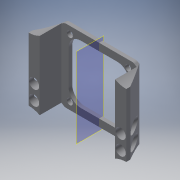
# Autodesk Inventor part: 30mm_fan_plus_radial
Saved by Autodesk Inventor 2019 (Build 230136000, 136)
## iProperties
Created: 2020-05-27
Part Number: 30mm_fan_plus_radial
Material: Generisch
Document SubType Name: Modeling
Designer: marc
Density: 1 g/cm^3
Appearance: Vorgabe
Author: marc
Autodesk Inventor part; units mm, degrees
ref_plane "YZ Plane" through (0, 0, 0) normal (1, 0, 0) x (0, 1, 0)
ref_plane "XZ Plane" through (0, 0, 0) normal (0, 1, 0) x (-1, 0, 0)
ref_plane "XY Plane" through (0, 0, 0) normal (0, 0, 1) x (1, 0, 0)
sketch "Skizze1" plane through (0, 0, 0) normal (0, 0, 1) x (1, 0, 0)
  arc A0 (-11.0395, 12.8) -> (-12.9605, 12.8) centre (-12, 12) ccw projected
  arc A1 (-12.9605, 11.2) -> (-11.0395, 11.2) centre (-12, 12) ccw projected
  arc A2 (-11.0395, -11.2) -> (-12.9605, -11.2) centre (-12, -12) ccw projected
  arc A3 (-12.9605, -12.8) -> (-11.0395, -12.8) centre (-12, -12) ccw projected
  arc A4 (12.9605, 12.8) -> (11.0395, 12.8) centre (12, 12) ccw projected
  arc A5 (11.0395, 11.2) -> (12.9605, 11.2) centre (12, 12) ccw projected
  arc A6 (11.0395, -12.8) -> (12.9605, -12.8) centre (12, -12) ccw projected
  arc A7 (12.9605, -11.2) -> (11.0395, -11.2) centre (12, -12) ccw projected
  line L0 (-13.5, 15) -> (13.5, 15)
  line L1 (15.5, 13) -> (15.5, -13)
  line L2 (13.5, -15) -> (-13.5, -15)
  line L3 (-15.5, -13) -> (-15.5, 13)
  arc A8 (-15.5, -13) -> (-13.5, -15) centre (-13.5, -13) ccw
  arc A9 (-13.5, 15) -> (-15.5, 13) centre (-13.5, 13) ccw
  arc A10 (15.5, 13) -> (13.5, 15) centre (13.5, 13) ccw
  arc A11 (13.5, -15) -> (15.5, -13) centre (13.5, -13) ccw
  line L4 (-7.5, -12) -> (7.5, -12)
  line L5 (12.5, -7) -> (12.5, 7)
  line L6 (7.5, 12) -> (-7.5, 12)
  line L7 (-12.5, 7) -> (-12.5, -7)
  arc A12 (-7.5, 12) -> (-12.5, 7) centre (-7.5, 7) ccw
  arc A13 (12.5, 7) -> (7.5, 12) centre (7.5, 7) ccw
  arc A14 (7.5, -12) -> (12.5, -7) centre (7.5, -7) ccw
  arc A15 (-12.5, -7) -> (-7.5, -12) centre (-7.5, -7) ccw
  circle A16 centre (-12, -12) radius 1.25
  circle A17 centre (12, 12) radius 1.25
  circle A18 centre (12, -12) radius 1.25
  circle A19 centre (-12, 12) radius 1.25
  point P0 (0, 0)
  point P1 (15.5, -15)
  point P2 (15.5, 15)
  point P3 (-15.5, -15)
  dimension "d0" = 31
  dimension "d1" = 30
  dimension "d2" = 3.5
  dimension "d3" = 3
  dimension "d4" = 2
  dimension "d5" = 5
  dimension "d6" = 5
  dimension "d7" = 3
  dimension "d8" = 3
  dimension "d9" = 3
  dimension "d10" = 3
  constraints: 16 end point, 16 point on circle, 16 tangent, 10 centre point, 7 equal radius, 6 point on line, 4 coincident, 4 parallel, 2 horizontal, 2 perpendicular, 6 other
  measures "d0" distance of point (15.5, -15) point (-15.5, -15)
  measures "d1" distance of point (15.5, 15) point (15.5, -15)
  measures "d2" distance from line of L3 A3.centre
  measures "d3" distance from line of L2 A2.centre
  measures "d4" radius of A8
  measures "d5" radius of A12
  measures "d6" radius of A13
  measures "d7" distance between parallel lines of L0 L6
  measures "d8" distance between parallel lines of L3 L7
  measures "d9" distance between parallel lines of L1 L5
  measures "d10" distance between parallel lines of L2 L4
extrude "Extrusion1" add sketch "Skizze1" along normal blind 1.5
sketch "Skizze2" plane through (15.5, -13, 0) normal (1, 0, 0) x (0, 0, -1)
  line L0 (0, 26) -> (-10.4, 26)
  line L1 (-10.4, 26) -> (-10.4, 0)
  line L2 (-10.4, 0) -> (0, 0)
  line L3 (0, 0) -> (0, 26)
  line L4 (0, 26) -> (-1.5, 26) projected
  point P0 (0, 13)
  dimension "d13" = 10.4
  constraints: 8 end point, 2 parallel, 1 coincident, 1 horizontal, 1 perpendicular
  measures "d13" distance of L1.end L2.end
extrude "Extrusion2" add sketch "Skizze2" along normal blind 4.6
chamfer "Fase1" distance 8.75 angle 25 1 edges at (20.1, 0, 0) measured on face at (20.1, 4.3333, 6.9333)
fillet "Rundung1" radius 9.75 1 edges at (15.5, -13, 0.75)
fillet "Rundung2" radius 9.75 1 edges at (15.5, 13, 0.75)
sketch "Skizze3" plane through (20.1, -13, 10.4) normal (0, 0, 1) x (1, 0, 0)
  line L0 (0, 26) -> (0, 0) projected
  line L1 (-4.6, -1.1307) -> (-4.6, 27.1307) projected
  point P0 (-20.1, 13)
  point P1 (-2.3, 9)
  point P2 (-2.3, 3)
  dimension "d21" = 2.3
  dimension "d22" = 4.6
  dimension "d23" = 3
  dimension "d24" = 6
  constraints: 1 vertical alignment
  measures "d21" distance from line of L0 point (-2.3, 3)
  measures "d22" distance between parallel lines of L0 L1
  measures "d23" vertical distance of L0.end point (-2.3, 3)
  measures "d24" distance of point (-2.3, 9) point (-2.3, 3)
hole "Bohrung1" at (17.8, -4, 10.4) at (17.8, -10, 10.4) direction (0, 0, -1) diameter 4.2 end through all
ref_plane "Arbeitsebene1" through (0, -13, 0) normal (-1, 0, 0) x (0, 0, 1)
mirror "Spiegeln1" about plane through (0, 0, 0) normal (1, 0, 0) of "Extrusion2", "Fase1", "Bohrung1"
fillet "Rundung3" radius 9.75 4 edges at (-15.5, 13, 5.95) (-15.5, 13, 0.75) (-15.5, -13, 0.75) (-15.5, -13, 5.95)
equation "\"d21\" = 0.5 * d22"
